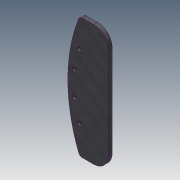
# Autodesk Inventor part: J005322
Saved by Autodesk Inventor 2015 SP1 (Build 190203100, 203)
## iProperties
Created: 2015-07-28
Material: STEEL, LOW CARBON (1008/1018/1020)
Vendor: HHMI: JRC - ID&F
Document SubType Name: Modeling
Designer: ARNOLDJ
Density: 7.85 g/cm^3
Appearance: Metal-Steel (Machined_00)
Mass: 65.5786 g
Surface Area: 61.1561 cm^2
Volume: 8.35396 cm^3
Part Number: J005322
Project: P-201804
Description: MBS LOCK PLATE ZT
RuleStatus: InUse
AfterDocSave0: file://Part Number Cleaner
LAB/DEPT: SVOBODA (LAB)
REQUESTING SCIENTIST: SVOBODA, KAREL
SURFACE ROUGHNESS: 63 Ra
DESIGN DEPARTMENT: HHMI: JRC - ID&F
SPECIAL FINISH: ELECTROLESS NICKEL (LOW PHOSPHOROUS) PER AMS-2405C, .001" THICK
ALTERED ITEM PART NUMBER: N/A
ALTERED ITEM VENDOR: N/A
ALTERED ITEM DESCRIPTION: N/A
Revision Number: -
Autodesk Inventor part; units mm, degrees
ref_plane "YZ Plane" through (0, 0, 0) normal (1, 0, 0) x (0, 1, 0)
ref_plane "XZ Plane" through (0, 0, 0) normal (0, 1, 0) x (-1, 0, 0)
ref_plane "XY Plane" through (0, 0, 0) normal (0, 0, 1) x (1, 0, 0)
sketch "Sketch1" plane through (0, 0, 0) normal (0, 0, 1) x (1, 0, 0)
  line L0 (0, 177.8) -> (0, -177.8) projected
  line L1 (-66.675, 0) -> (288.925, 0) projected
  line L2 (15.875, -47.625) -> (-15.875, -47.625)
  line L3 (-15.875, -47.625) -> (-15.875, 47.625)
  line L4 (-15.875, 47.625) -> (15.875, 47.625)
  line L5 (15.875, 47.625) -> (15.875, -47.625)
  line L6 (0, 0) -> (0, 35.5411)
  circle A0 centre (71.6788, 0) radius 60.6679 construction
  circle A1 centre (71.6788, 0) radius 56.8579 construction
  circle A2 centre (71.6788, 0) radius 83.5279 construction
  line L7 (0, 47.625) -> (-15.875, 34.925) construction
  circle A3 centre (111.125, 0) radius 127
  point P0 (-10.795, 9.525)
  point P1 (-10.795, -9.525)
  point P2 (-6.985, 25.4)
  point P3 (-6.985, -25.4)
  dimension "d0" = 31.75
  dimension "d15" = 47.625
  dimension "d16" = 47.625
  dimension "d20" = 0
  dimension "d21" = 71.6788
  dimension "d22" = 121.3358
  dimension "d23" = 3.81
  dimension "d25" = 22.86
  dimension "d26" = 15.875
  dimension "d27" = 12.7
  dimension "d28" = 9.525
  dimension "d29" = 9.525
  dimension "d32" = 8.89
  dimension "d33" = 5.08
  dimension "d34" = 15.875
  dimension "d35" = 15.875
  dimension "d36" = 254
  dimension "d37" = 127
  constraints: 12 end point, 4 centre point, 2 midpoint, 2 parallel, 2 point on line, 2 vertical alignment, 1 coincident, 1 horizontal, 1 perpendicular, 1 other
  measures "d0" distance of L3.end L4.end
  measures "d15" distance between parallel lines of L1 L4
  measures "d16" distance between parallel lines of L1 L2
  measures "d20" distance from line of L1 point (71.679, 0)
  measures "d21" distance from line of point (71.679, 0) L0
  measures "d22" diameter of A0
  measures "d23" radial gap between concentric circles of A1 A0
  measures "d25" radial gap between concentric circles of A0 A2
  measures "d26" distance from line of L7.start L3
  measures "d27" distance from line of L7.end L4
  measures "d28" distance from line of point (-10.795, 9.525) L1
  measures "d29" distance from line of L1 point (-10.795, -9.525)
  measures "d32" distance from line of L3 point (-6.985, 25.4)
  measures "d33" distance from line of L3 point (-10.795, 9.525)
  measures "d34" vertical distance of point (-10.795, 9.525) point (-6.985, 25.4)
  measures "d35" vertical distance of point (-6.985, -25.4) point (-10.795, -9.525)
  measures "d36" diameter of A3
  measures "d37" distance from line of L3 A3.centre
extrude "Extrusion1" add sketch "Sketch1" along normal blind 3.175 contours L1 A3 L4 L0 | L1 L5 L2 L0 | L0 L2 A3 L1 | L0 L4 L5 L1 | A3 L2 L3 | L3 L4 A3
hole "Hole1" at (-10.795, 9.525, 0) at (-10.795, -9.525, 0) at (-6.985, 25.4, 0) at (-6.985, -25.4, 0) direction (0, 0, 1) diameter 3.2512 end through all countersink diameter 6.35 countersink angle 90
fillet "Fillet1" radius 11.43 2 edges at (15.875, 47.625, 1.5875) (15.875, -47.625, 1.5875)
sketch "Sketch2" plane through (0, 0, 0) normal (0, 0, 1) x (1, 0, 0)
  circle A0 centre (111.125, 0) radius 127 projected
  line L0 (4.445, 47.625) -> (-15.875, 47.625) projected
  line L1 (-15.875, -47.625) -> (4.445, -47.625) projected
  line L2 (-15.875, 47.625) -> (-15.875, -47.625) projected
  arc A1 (-6.6072, 47.625) -> (-6.6072, -47.625) centre (111.125, 0) ccw
  line L3 (-6.6072, 47.625) -> (-15.875, 47.625)
  line L4 (-15.875, 0) -> (-15.875, -47.625)
  line L5 (-15.875, -47.625) -> (-6.6072, -47.625)
  line L6 (-15.875, 47.625) -> (-15.875, 0)
  point P0 (0, 0)
  constraints: 8 end point, 3 point on circle, 3 tangent, 2 collinear, 2 point on line, 1 centre point, 1 coincident, 1 midpoint, 1 perpendicular
extrude "Extrusion2" cut sketch "Sketch2" along normal blind 25.4 contours A0 L2 L0 | L1 L2 A0
fillet "Fillet2" radius 3.175 2 edges at (-6.6072, 47.625, 1.5875) (-6.6072, -47.625, 1.5875)
equation "\"d26\" = 0.5 * d0"
body "Solid1"
